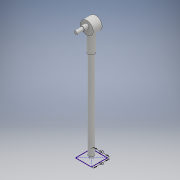
# Autodesk Inventor part: ラックアンドピニオンの左右の棒
Saved by Autodesk Inventor 2018 (Build 220112000, 112)
## iProperties
Created: 2017-09-10
Part Number: ラックアンドピニオンの左右の棒
Material: 一般
Document SubType Name: Modeling
Designer: Kenta
Density: 1 g/cm^3
Appearance: 既定
Author: Kenta
Autodesk Inventor part; units mm, degrees
ref_plane "YZ Plane" through (0, 0, 0) normal (1, 0, 0) x (0, 1, 0)
ref_plane "XZ Plane" through (0, 0, 0) normal (0, 1, 0) x (-1, 0, 0)
ref_plane "XY Plane" through (0, 0, 0) normal (0, 0, 1) x (1, 0, 0)
sketch "スケッチ1" plane through (0, 0, 0) normal (0, 0, 1) x (1, 0, 0)
  circle A0 centre (0, 0) radius 8
  dimension "d0" = 16
  constraints: 1 centre point, 1 coincident
  measures "d0" diameter of A0
extrude "押し出し1" add sketch "スケッチ1" along normal blind 288
sketch "スケッチ2" plane through (0, 0, 0) normal (0, 0, -1) x (-1, 0, 0)
  point P0 (0, 0)
  point P1 (0, 0)
  constraints: 1 coincident
fillet "フィレット1" radius 8 1 edges at (-8, 0, 0)
sketch "スケッチ3" plane through (0, 0, 288) normal (0, 0, 1) x (1, 0, 0)
  circle A0 centre (0, 0) radius 10.5
  dimension "d4" = 21
  constraints: 1 centre point, 1 coincident
  measures "d4" diameter of A0
extrude "押し出し2" add sketch "スケッチ3" along normal blind 82
sketch "スケッチ4" plane through (0, 0, 0) normal (0, 1, 0) x (-1, 0, 0)
  circle A0 centre (0, 361.9107) radius 20
  point P0 (0, 0)
  dimension "d7" = 40
  constraints: 1 centre point
  measures "d7" diameter of A0
extrude "押し出し3" add sketch "スケッチ4" along normal mid plane 28
ref_plane "作業平面1" through (0, 0, 348) normal (0, 0, -1) x (-1, 0, 0)
sketch "スケッチ5" plane through (0, 0, 348) normal (0, 0, -1) x (-1, 0, 0)
  line L0 (10.5, 15) -> (-10.5, 15)
  line L1 (-10.5, 15) -> (-10.5, -15)
  line L2 (-10.5, -15) -> (10.5, -15)
  line L3 (10.5, -15) -> (10.5, 15)
  line L4 (10.5, 15) -> (-10.5, -15) construction
  line L5 (-10.5, 15) -> (10.5, -15) construction
  point P0 (0, 0)
  dimension "d11" = 21
  dimension "d12" = 30
  constraints: 12 end point, 2 midpoint, 2 parallel, 1 horizontal, 1 perpendicular
  measures "d11" distance of L2.end L1.end
  measures "d12" distance of L1.end L0.end
ref_plane "作業平面2" through (10.5, -15, 348) normal (0, 0.9986295, 0.052336) x (-1, 0, 0)
sketch "スケッチ8" plane through (10.5, -15, 348) normal (0, 0.9986295, 0.052336) x (-1, 0, 0)
  circle A0 centre (10.5, 19.2998) radius 6.5
  point P0 (10.5, -348.3081)
  dimension "d14" = 13
  constraints: 2 coincident, 1 centre point
  measures "d14" diameter of A0
extrude "押し出し4" add sketch "スケッチ8" along normal mid plane 24
sketch "スケッチ9" plane through (0, -27.9936, 366.6453) normal (0, -0.9986295, -0.052336) x (1, 0, 0)
  circle A0 centre (0, 0) radius 5
  point P0 (0, -367.6079)
  dimension "d17" = 10
  constraints: 1 centre point
  measures "d17" diameter of A0
extrude "押し出し5" add sketch "スケッチ9" along normal blind 21
sketch "スケッチ11" plane through (0, 0, 0) normal (0, 0, 1) x (1, 0, 0)
  line L0 (-25, -25) -> (25, -25)
  line L1 (25, -25) -> (25, 25)
  line L2 (25, 25) -> (-25, 25)
  line L3 (-25, 25) -> (-25, -25)
  line L4 (-25, -25) -> (25, 25) construction
  line L5 (25, -25) -> (-25, 25) construction
  point P0 (0, 0)
  dimension "d23" = 50
  dimension "d24" = 50
  constraints: 12 end point, 2 midpoint, 2 parallel, 1 horizontal, 1 perpendicular
  measures "d23" distance of L2.end L1.end
  measures "d24" distance of L1.end L0.end
